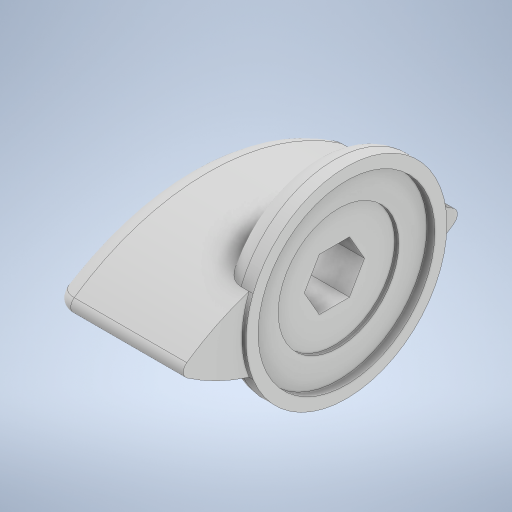
# Autodesk Inventor part: Parte5
Saved by Autodesk Inventor 2024 (Build 280153000, 153)
## iProperties
Created: 2023-12-18
Part Number: Parte5
Material: Generico
Document SubType Name: Modeling
Designer: cecca
Density: 1 g/cm^3
Appearance: Default
Author: cecca
Autodesk Inventor part; units mm, degrees
ref_plane "YZ Plane" through (0, 0, 0) normal (1, 0, 0) x (0, 1, 0)
ref_plane "XZ Plane" through (0, 0, 0) normal (0, 1, 0) x (-1, 0, 0)
ref_plane "XY Plane" through (0, 0, 0) normal (0, 0, 1) x (1, 0, 0)
sketch "Schizzo1" plane through (0, 0, 0) normal (1, 0, 0) x (0, 1, 0)
  circle A0 centre (0, 0) radius 25
  dimension "d0" = 50
  constraints: 1 centre point, 1 coincident
  measures "d0" diameter of A0
extrude "Estrusione1" add sketch "Schizzo1" along normal blind 8
sketch "Schizzo2" plane through (8, 0, 0) normal (1, 0, 0) x (0, 0, -1)
  line L0 (0, 0) -> (46.834, 0) construction
  circle A0 centre (-5.4966, -46.5103) radius 58.5105
  line L1 (0, 0) -> (-62.129, 0)
  circle A1 centre (-5.4966, 46.5103) radius 58.5105
  circle A2 centre (0, 0) radius 2.5
  point P0 (-40.9969, 0)
  point P1 (30.0036, 0)
  dimension "d6" = 5
  constraints: 4 end point, 3 centre point, 2 horizontal, 1 coincident, 1 symmetric about line, 1 other
  measures "d6" diameter of A2
extrude "Estrusione2" add sketch "Schizzo2" against normal blind 34 contours A1 A0 picked at (-10.8272, 0)
fillet "Raccordo1" radius 2 2 edges at (-9, 0, 40.9969) (-9, 0, -30.0036)
fillet "Raccordo2" radius 5 4 edges at (-26, 0, 39.5938) (-26, 12.0002, 5.4966) (-26, 0, -28.6005) (-26, -12.0002, 5.4966)
fillet "Raccordo3" radius 5 2 edges at (0, -24.8272, -2.9341) (0, 24.8272, -2.9341)
sketch "Schizzo4" plane through (8, 0, 0) normal (1, 0, 0) x (0, 0, -1)
  circle A0 centre (0, 0) radius 2.5 projected
  circle A1 centre (0, 0) radius 25
  line L0 (-23.2272, -9.2464) -> (-45.7122, -17.0053)
  line L1 (-45.7122, -17.0053) -> (-45.7122, 23.1523)
  line L2 (-45.7122, 23.1523) -> (-23.2272, 9.2464)
  line L3 (24.7388, -3.6043) -> (36.4668, -10.8575)
  line L4 (36.4668, -10.8575) -> (36.4668, 6.498)
  line L5 (36.4668, 6.498) -> (24.7388, 3.6043)
  constraints: 12 end point, 4 point on circle, 2 parallel, 1 centre point, 1 coincident, 1 vertical
extrude "Estrusione4" cut sketch "Schizzo4" against normal blind 1 contours A1 L5 L4 L3 | A1 L0 L1 L2
sketch "Schizzo5" plane through (8, 0, 0) normal (1, 0, 0) x (0, 0, -1)
  line L0 (3.7525, 6.5) -> (-3.7525, 6.5)
  line L1 (-3.7525, -6.5) -> (3.7525, -6.5)
  line L2 (-7.5055, 0) -> (-3.7525, 6.5)
  line L3 (-3.7525, -6.5) -> (-7.5055, 0)
  line L4 (7.5055, 0) -> (3.7525, 6.5)
  line L5 (3.7525, -6.5) -> (7.5055, 0)
  point P0 (0, 0)
  constraints: 12 end point
extrude "Estrusione5" cut sketch "Schizzo5" against normal blind 15
sketch "Schizzo6" plane through (8, 0, 0) normal (1, 0, 0) x (0, 0, -1)
  circle A0 centre (0, 0) radius 2.5 projected
  circle A1 centre (0, 0) radius 22
  dimension "d23" = 44
  constraints: 1 centre point, 1 coincident
  measures "d23" diameter of A1
extrude "Estrusione6" cut sketch "Schizzo6" against normal blind 2
sketch "Schizzo7" plane through (6, 0, 0) normal (1, 0, 0) x (0, 0, -1)
  circle A0 centre (0, 0) radius 15
  dimension "d26" = 30
  constraints: 1 centre point, 1 coincident
  measures "d26" diameter of A0
extrude "Estrusione7" cut sketch "Schizzo7" against normal blind 1
